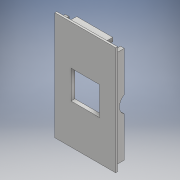
# Autodesk Inventor part: hull_cover
Saved by Autodesk Inventor 2018 (Build 220112000, 112)
## iProperties
Created: 2018-01-11
Part Number: hull_cover
Material: Generic
Document SubType Name: Modeling
Designer: erwin
Density: 1 g/cm^3
Appearance: Default
Author: erwin
Autodesk Inventor part; units mm, degrees
ref_plane "YZ Plane" through (0, 0, 0) normal (1, 0, 0) x (0, 1, 0)
ref_plane "XZ Plane" through (0, 0, 0) normal (0, 1, 0) x (-1, 0, 0)
ref_plane "XY Plane" through (0, 0, 0) normal (0, 0, 1) x (1, 0, 0)
sketch "Sketch1" plane through (0, 0, 0) normal (0, 1, 0) x (-1, 0, 0)
  line L0 (16, -28.5) -> (-16, -28.5)
  line L1 (-16, -28.5) -> (-16, 28.5)
  line L2 (-16, 28.5) -> (16, 28.5)
  line L3 (16, 28.5) -> (16, -28.5)
  line L4 (16, -28.5) -> (-16, 28.5) construction
  line L5 (-16, -28.5) -> (16, 28.5) construction
  point P0 (0, 0)
  dimension "d0" = 32
  dimension "d1" = 57
  constraints: 12 end point, 2 midpoint, 2 parallel, 1 horizontal, 1 perpendicular
  measures "d0" distance of L1.end L2.end
  measures "d1" distance of L0.end L1.end
extrude "Extrusion1" add sketch "Sketch1" along normal blind 1
sketch "Sketch2" plane through (0, 1, 0) normal (0, 1, 0) x (1, 0, 0)
  line L0 (-9.5, -27.5) -> (9.5, -27.5)
  line L1 (15.5, -25.5) -> (15.5, 25.5)
  line L2 (9.5, 27.5) -> (-9.5, 27.5)
  line L3 (-15.5, 25.5) -> (-15.5, -25.5)
  line L4 (-15.5, -27.5) -> (15.5, 27.5) construction
  line L5 (15.5, -27.5) -> (-15.5, 27.5) construction
  line L6 (13.5, -25.5) -> (13.5, 25.5)
  line L7 (-13.5, 25.5) -> (-13.5, -25.5)
  line L8 (-16, -28.5) -> (16, -28.5) projected
  line L9 (-9.5, -28.4306) -> (-9.5, -25.5)
  line L10 (9.5, 25.5) -> (9.5, 27.5)
  line L11 (-9.5, -16.8548) -> (-9.5, 16.8548)
  line L12 (-9.5, 25.5) -> (-9.5, 28.5928)
  line L13 (9.5, -28.5) -> (9.5, -25.5)
  line L14 (9.5, -16.8548) -> (9.5, 16.8548)
  line L15 (13.5, -25.5) -> (15.5, -25.5)
  line L16 (15.5, 25.5) -> (13.5, 25.5)
  line L17 (9.5, 25.5) -> (-9.5, 25.5)
  line L18 (-13.5, 25.5) -> (-15.5, 25.5)
  line L19 (-15.5, -25.5) -> (-13.5, -25.5)
  line L20 (-9.5, -25.5) -> (9.5, -25.5)
  point P0 (0, 0)
  dimension "d4" = 31
  dimension "d5" = 55
  dimension "d6" = 2
  constraints: 40 end point, 12 parallel, 8 point on line, 7 perpendicular, 3 vertical, 2 midpoint, 1 horizontal
  measures "d4" distance of L5.end L4.end
  measures "d5" distance of L4.end L5.start
  measures "d6" distance between parallel lines of L3 L7
extrude "Extrusion2" add sketch "Sketch2" along normal blind 4
sketch "Sketch3" plane through (15.5, 1, 25.5) normal (1, 0, 0) x (0, 0, -1)
  circle A0 centre (25.5, 6.5) radius 5
  line L0 (-3, 0) -> (54, 0) projected
  point P0 (25.5, -1)
  dimension "d11" = 10
  dimension "d12" = 6.5
  constraints: 1 centre point
  measures "d11" diameter of A0
  measures "d12" distance from line of L0 A0.centre
extrude "Extrusion3" cut sketch "Sketch3" against normal through all
sketch "Sketch4" plane through (0, 0, 0) normal (0, -1, 0) x (1, 0, 0)
  line L0 (7.5, -7.5) -> (-7.5, -7.5)
  line L1 (-7.5, -7.5) -> (-7.5, 7.5)
  line L2 (-7.5, 7.5) -> (7.5, 7.5)
  line L3 (7.5, 7.5) -> (7.5, -7.5)
  line L4 (7.5, -7.5) -> (-7.5, 7.5) construction
  line L5 (-7.5, -7.5) -> (7.5, 7.5) construction
  point P0 (0, 0)
  dimension "d15" = 15
  dimension "d16" = 15
  constraints: 12 end point, 2 midpoint, 2 parallel, 1 horizontal, 1 perpendicular
  measures "d15" distance of L1.end L2.end
  measures "d16" distance of L0.end L1.end
extrude "Extrusion4" cut sketch "Sketch4" against normal through all
sketch "Sketch5" plane through (0, 1, 0) normal (0, 1, 0) x (1, 0, 0)
  line L0 (7.5, 7.5) -> (7.5, -7.5) projected
  line L1 (7.5, -7.5) -> (-7.5, -7.5) projected
  line L2 (-7.5, -7.5) -> (-7.5, 7.5) projected
  line L3 (-7.5, 7.5) -> (7.5, 7.5) projected
  line L4 (-13.5, -25.5) -> (-15.5, -25.5) projected
  line L5 (-15.5, -25.5) -> (-15.5, 25.5) projected
  line L6 (-15.5, 25.5) -> (-13.5, 25.5) projected
  line L7 (-13.5, 25.5) -> (-13.5, -25.5) projected
  line L8 (9.5, -27.5) -> (-9.5, -27.5) projected
  line L9 (-9.5, -27.5) -> (-9.5, -25.5) projected
  line L10 (-9.5, -25.5) -> (9.5, -25.5) projected
  line L11 (9.5, -25.5) -> (9.5, -27.5) projected
  line L12 (9.5, 27.5) -> (9.5, 25.5) projected
  line L13 (9.5, 25.5) -> (-9.5, 25.5) projected
  line L14 (-9.5, 25.5) -> (-9.5, 27.5) projected
  line L15 (-9.5, 27.5) -> (9.5, 27.5) projected
  line L16 (13.5, 25.5) -> (15.5, 25.5) projected
  line L17 (15.5, 25.5) -> (15.5, -25.5) projected
  line L18 (15.5, -25.5) -> (13.5, -25.5) projected
  line L19 (13.5, -25.5) -> (13.5, 25.5) projected
  line L20 (16, 28.5) -> (-16, 28.5) projected
  line L21 (-16, 28.5) -> (-16, -28.5) projected
  line L22 (-16, -28.5) -> (16, -28.5) projected
  line L23 (16, -28.5) -> (16, 28.5) projected
  line L24 (-8.5, -8.5) -> (8.5, -8.5)
  line L25 (8.5, -8.5) -> (8.5, 8.5)
  line L26 (8.5, 8.5) -> (-8.5, 8.5)
  line L27 (-8.5, 8.5) -> (-8.5, -8.5)
  point P0 (0, 0)
  dimension "d19" = 1
  constraints: 8 end point, 3 other
  measures "d19" distance between parallel lines of L1 L24
extrude "Extrusion5" add sketch "Sketch5" along normal blind 1 contours L27 L26 L25 L24
body "Solid1"
